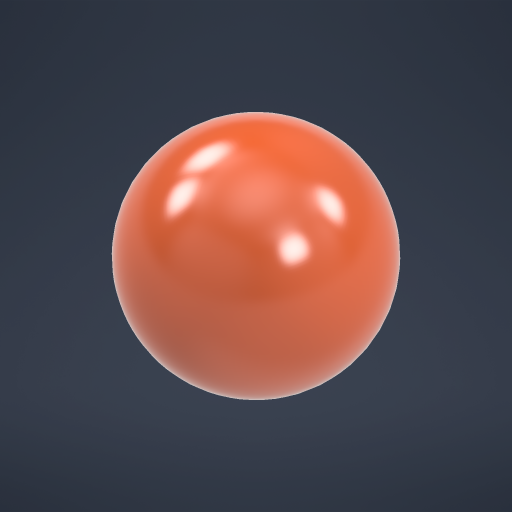
# Autodesk Inventor part: Ball
Saved by Autodesk Inventor 2024.2 (Build 282272000, 272)
## iProperties
Created: 2023-12-21
Part Number: Ball
Material: 一般
Document SubType Name: Modeling
Designer: Hanaoka
Density: 1 g/cm^3
Appearance: 既定
Author: Hanaoka
Autodesk Inventor part; units mm, degrees
ref_plane "YZ Plane" through (0, 0, 0) normal (1, 0, 0) x (0, 1, 0)
ref_plane "XZ Plane" through (0, 0, 0) normal (0, 1, 0) x (-1, 0, 0)
ref_plane "XY Plane" through (0, 0, 0) normal (0, 0, 1) x (1, 0, 0)
sketch "スケッチ1" plane through (0, 0, 0) normal (0, 0, 1) x (1, 0, 0)
  arc A0 (0, -21) -> (0, 21) centre (0, 0) ccw
  line L0 (0, 21) -> (0, -21)
  line L1 (0, -29.4) -> (0, 29.4) projected
  dimension "d0" = 21
  constraints: 2 end point, 2 point on circle, 2 point on line, 1 centre point, 1 coincident
  measures "d0" radius of A0
revolve "回転1" add sketch "スケッチ1" angle 360 about axis through (0, -10, 0) along (0, 1, 0)
